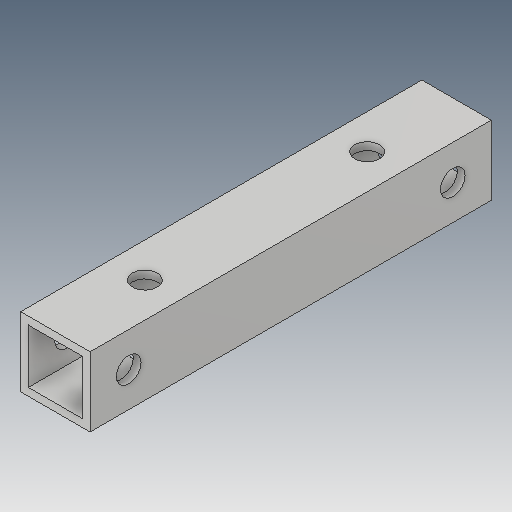
# Autodesk Inventor part: 型
Saved by Autodesk Inventor 2019.4 (Build 234330000, 330)
## iProperties
Created: 2019-06-27
Part Number: 型
Material: アルミニウム 2014-T6
Document SubType Name: Modeling
Designer: 長谷川翔一
Density: 2.78927 g/cm^3
Appearance: サテン
Mass: 4.01655 g
Surface Area: 29.44 cm^2
Volume: 1.44 cm^3
Author: 長谷川翔一
Autodesk Inventor part; units mm, degrees
ref_plane "YZ Plane" through (0, 0, 0) normal (1, 0, 0) x (0, 1, 0)
ref_plane "XZ Plane" through (0, 0, 0) normal (0, 1, 0) x (-1, 0, 0)
ref_plane "XY Plane" through (0, 0, 0) normal (0, 0, 1) x (1, 0, 0)
sketch "スケッチ1" plane through (0, 0, 0) normal (0, 0, 1) x (1, 0, 0)
  line L0 (4.5, -4.5) -> (-4.5, -4.5)
  line L1 (-4.5, -4.5) -> (-4.5, 4.5)
  line L2 (-4.5, 4.5) -> (4.5, 4.5)
  line L3 (4.5, 4.5) -> (4.5, -4.5)
  line L4 (4.5, -4.5) -> (-4.5, 4.5) construction
  line L5 (-4.5, -4.5) -> (4.5, 4.5) construction
  line L6 (3.5, 3.5) -> (-3.5, 3.5)
  line L7 (-3.5, 3.5) -> (-3.5, -3.5)
  line L8 (-3.5, -3.5) -> (3.5, -3.5)
  line L9 (3.5, -3.5) -> (3.5, 3.5)
  point P0 (0, 0)
  dimension "d0" = 9
  dimension "d1" = 9
  dimension "d2" = 1
  constraints: 20 end point, 4 parallel, 2 midpoint, 2 perpendicular, 1 horizontal, 3 other
  measures "d0" distance of L1.end L2.end
  measures "d1" distance of L0.end L1.end
  measures "d2" distance between parallel lines of L2 L6
extrude "押し出し1" add sketch "スケッチ1" along normal blind 52
sketch "スケッチ3" plane through (4.5, -4.5, 0) normal (1, 0, 0) x (0, 0, -1)
  line L0 (0, 9) -> (0, 0) projected
  line L1 (0, 9) -> (-52, 9) projected
  line L2 (-52, 0) -> (-52, 9) projected
  line L3 (0, 0) -> (-52, 0) projected
  line L4 (-52, 4.5) -> (0, 4.5) construction
  line L5 (-26, 4.5) -> (-26, 9) construction
  circle A0 centre (-47, 4.5) radius 1.6
  circle A1 centre (-5, 4.5) radius 1.6
  dimension "d9" = 3.2
  dimension "d10" = 5
  constraints: 4 end point, 3 midpoint, 2 centre point, 1 horizontal, 1 point on line, 1 symmetric about line, 1 other
  measures "d9" diameter of A0
  measures "d10" distance from line of A0.centre L2
extrude "押し出し3" cut sketch "スケッチ3" against normal through all contours A0 | A1
sketch "スケッチ4" plane through (-4.5, -4.5, 0) normal (0, -1, 0) x (1, 0, 0)
  line L0 (9, 0) -> (0, 0) projected
  line L1 (9, 0) -> (9, 52) projected
  line L2 (0, 52) -> (9, 52) projected
  line L3 (0, 0) -> (0, 52) projected
  line L4 (9, 48.6) -> (9, 45.4) projected
  line L5 (8, 45.4) -> (8, 48.6) projected
  line L6 (0, 48.6) -> (0, 45.4) projected
  line L7 (1, 48.6) -> (1, 45.4) projected
  line L8 (9, 6.6) -> (9, 3.4) projected
  line L9 (8, 3.4) -> (8, 6.6) projected
  line L10 (1, 6.6) -> (1, 3.4) projected
  line L11 (4.5, 52) -> (4.5, 0) construction
  line L12 (9, 45.4) -> (0, 45.4)
  circle A0 centre (4.5, 40.4) radius 1.6
  line L13 (9, 26) -> (0, 26) construction
  circle A1 centre (4.5, 11.6) radius 1.6
  dimension "d13" = 3.2
  dimension "d14" = 5
  dimension "d15" = 4.5
  constraints: 6 end point, 3 midpoint, 2 centre point, 1 perpendicular, 1 point on line, 1 symmetric about line, 1 vertical, 1 other
  measures "d13" diameter of A0
  measures "d14" distance from line of A0.centre L12
  measures "d15" distance from line of L1 A0.centre
extrude "押し出し4" cut sketch "スケッチ4" against normal through all contours A0 | A1
